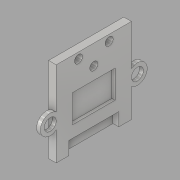
# Autodesk Inventor part: Pi cCam Mount
Saved by Autodesk Inventor 2017 (Build 210142000, 142)
## iProperties
Created: 2016-12-08
Part Number: Pi cCam Mount
Material: Aluminum 6061-AHC
Document SubType Name: Modeling
Designer: qupec
Density: 2.7 g/cm^3
Appearance: Aluminum - Dark
Mass: 8.38024 g
Surface Area: 29.6366 cm^2
Volume: 3.10379 cm^3
Author: qupec
Autodesk Inventor part; units mm, degrees
ref_plane "YZ Plane" through (0, 0, 0) normal (1, 0, 0) x (0, 1, 0)
ref_plane "XZ Plane" through (0, 0, 0) normal (0, 1, 0) x (-1, 0, 0)
ref_plane "XY Plane" through (0, 0, 0) normal (0, 0, 1) x (1, 0, 0)
sketch "Sketch2" plane through (0, 0, 0) normal (1, 0, 0) x (0, 1, 0)
  line L0 (12, 15.675) -> (-12, 15.675)
  line L1 (-12, 15.675) -> (-12, -15.675)
  line L2 (-12, -15.675) -> (12, -15.675)
  line L3 (12, -15.675) -> (12, 15.675)
  point P0 (0, 0)
  dimension "d4" = 24
  dimension "d5" = 31.35
  dimension "d6" = 15.675
  dimension "d7" = 12
  constraints: 8 end point, 2 parallel, 1 horizontal, 1 perpendicular
  measures "d4" distance of L0.start L0.end
  measures "d5" distance of L2.end L0.start
  measures "d6" distance from line of point (0, 0) L0
  measures "d7" distance from line of point (0, 0) L1
extrude "Extrusion1" add sketch "Sketch2" along normal blind 3.175
sketch "Sketch3" plane through (3.175, 0, 0) normal (1, 0, 0) x (0, 0, -1)
  line L0 (-15.675, -12) -> (15.675, -12) projected
  line L1 (-10.4, -12) -> (10.4, -12)
  line L2 (10.4, -12) -> (10.4, -6.5)
  line L3 (10.4, -6.5) -> (-10.4, -6.5)
  line L4 (-10.4, -6.5) -> (-10.4, -12)
  point P0 (0, 0)
  dimension "d16" = 20.8
  dimension "d17" = 10.4
  dimension "d18" = 5.5
  constraints: 8 end point, 2 parallel, 1 horizontal, 1 perpendicular, 1 point on line
  measures "d16" distance of L2.end L3.end
  measures "d17" distance from line of point (0, 0) L4
  measures "d18" distance of L3.end L1.start
extrude "Extrusion2" cut sketch "Sketch3" against normal blind 2.4
sketch "Sketch4" plane through (3.175, 0, 0) normal (1, 0, 0) x (0, 0, -1)
  line L0 (-8.85, 10) -> (8.85, 10)
  line L1 (8.85, 10) -> (8.85, -1.6)
  line L2 (8.85, -1.6) -> (-8.85, -1.6)
  line L3 (-8.85, -1.6) -> (-8.85, 10)
  line L4 (-10.4, -6.5) -> (10.4, -6.5) projected
  line L5 (10.4, -12) -> (-10.4, -12) projected
  point P0 (0, 4.2)
  dimension "d21" = 17.7
  dimension "d22" = 8.85
  dimension "d23" = 5.8
  dimension "d24" = 11.6
  dimension "d27" = 10.4
  constraints: 8 end point, 2 parallel, 1 horizontal, 1 perpendicular
  measures "d21" distance of L0.start L0.end
  measures "d22" distance from line of L3 point (0, 4.2)
  measures "d23" distance from line of point (0, 4.2) L2
  measures "d24" distance of L2.end L0.start
  measures "d27" distance between parallel lines of L5 L2
extrude "Extrusion3" cut sketch "Sketch4" against normal blind 1.3
sketch "Sketch5" plane through (3.175, 0, 0) normal (1, 0, 0) x (0, 0, -1)
  circle A0 centre (-10.65, 10.9) radius 0.8411
  circle A1 centre (10.65, 10.9) radius 0.8411
  line L0 (-15.675, 12) -> (-15.675, -12) projected
  line L1 (15.675, 12) -> (-15.675, 12) projected
  line L2 (15.675, -12) -> (15.675, 12) projected
  line L3 (8.85, 10) -> (8.85, -1.6) projected
  line L4 (-8.85, 10) -> (8.85, 10) projected
  point P0 (0, 0)
  dimension "d31" = 1.6822
  dimension "d33" = 1.6822
  dimension "d60" = 1.8
  dimension "d62" = 0.9
  dimension "d67" = 0.9
  dimension "d68" = 1.8
  constraints: 2 centre point
  measures "d31" diameter of A0
  measures "d33" diameter of A1
  measures "d60" distance from line of A1.centre L3
  measures "d62" vertical distance of L3.start A1.centre
  measures "d67" distance from line of L4 A0.centre
  measures "d68" horizontal distance of L4.start A0.centre
extrude "Extrusion7" [suppressed]
sketch "Sketch10" plane through (3.175, 0, 0) normal (1, 0, 0) x (0, 0, -1)
  circle A0 centre (-18.175, 3.175) radius 2.5
  line L0 (-15.675, 12) -> (-15.675, -12) construction
  arc A1 (-15.675, 6.4088) -> (-15.675, -0.0588) centre (-18.175, 3.175) ccw
  line L1 (0, 13.5875) -> (0, -23.7475) construction
  circle A2 centre (18.175, 3.175) radius 2.5
  arc A3 (15.675, -0.0588) -> (15.675, 6.4088) centre (18.175, 3.175) ccw
  line L2 (15.675, 12) -> (-15.675, 12) projected
  line L3 (-15.675, 6.4088) -> (-15.675, -0.0588)
  line L4 (15.675, -12) -> (15.675, 12) projected
  line L5 (15.675, 6.4088) -> (15.675, -0.0588)
  point P0 (0, 0)
  dimension "d73" = 8.175
  dimension "d74" = 5
  dimension "d80" = 24
  dimension "d81" = 15.175
  constraints: 6 end point, 4 centre point, 4 point on circle, 4 point on line, 3 symmetric about line, 2 coincident, 1 tangent, 1 vertical, 2 other
  measures "d73" diameter of A1
  measures "d74" diameter of A0
  measures "d80" distance of L0.start L0.end
  measures "d81" vertical distance of L0.end A0.centre
extrude "Extrusion13" add sketch "Sketch10" against normal blind 1.5875
sketch "Sketch12" plane through (0, 12, 15.675) normal (0, 1, 0) x (1, 0, 0)
  line L0 (0, 31.35) -> (0, 0) projected
  line L1 (0, 0) -> (3.175, 0) projected
  line L2 (3.175, 31.35) -> (3.175, 0) projected
  line L3 (0, 31.35) -> (3.175, 31.35) projected
  point P0 (0, 15.675)
extrude "Extrusion14" add sketch "Sketch12" along normal blind 11.43
sketch "Sketch13" plane through (0, 0, 0) normal (-1, 0, 0) x (0, 0, 1)
  circle A0 centre (-6.3786, 20.89) radius 1.6764
  circle A1 centre (6.3786, 20.89) radius 1.6764
  line L0 (-15.675, 23.43) -> (15.675, 23.43) projected
  line L1 (-15.675, -12) -> (-15.675, 23.43) projected
  line L2 (15.675, 23.43) -> (15.675, -12) projected
  circle A2 centre (0, 15.175) radius 1.6764
  point P0 (0, 0)
  dimension "d92" = 3.3528
  dimension "d93" = 3.3528
  dimension "d94" = 2.54
  dimension "d95" = 9.2964
  dimension "d96" = 9.2964
  dimension "d97" = 2.54
  dimension "d98" = 3.3528
  dimension "d99" = 8.255
  dimension "d100" = 31.35
  dimension "d101" = 15.675
  constraints: 3 centre point
  measures "d92" diameter of A0
  measures "d93" diameter of A1
  measures "d94" distance from line of L0 A0.centre
  measures "d95" distance from line of L1 A0.centre
  measures "d96" distance from line of L2 A1.centre
  measures "d97" distance from line of L0 A1.centre
  measures "d98" diameter of A2
  measures "d99" distance from line of L0 A2.centre
  measures "d100" distance of L0.start L0.end
  measures "d101" distance from line of L1 A2.centre
extrude "Extrusion15" cut sketch "Sketch13" against normal through all
equation "\"d6\" = 0.5 * d5"
equation "\"d7\" = 0.5 * d4"
equation "\"d17\" = 0.5 * d16"
equation "\"d22\" = 0.5 * d21"
equation "\"d23\" = 0.5 * d24"
equation "\"d31\" = d30"
equation "\"d33\" = d30"
equation "\"d67\" = d62"
equation "\"d68\" = d60"
equation "\"d93\" = d92"
equation "\"d96\" = d95"
equation "\"d98\" = d92"
equation "\"d101\" = 0.5 * d100"
equation "\"d30\" = 1.682224"
body "Solid1"
